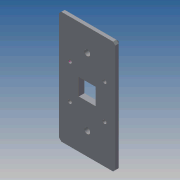
# Autodesk Inventor part: nema y axis cover
Saved by Autodesk Inventor 2015 (Build 190159000, 159)
## iProperties
Created: 2015-10-11
Part Number: nema y axis cover
Material: Generic
Document SubType Name: Modeling
Designer: Solomon
Density: 1 g/cm^3
Appearance: Default
Author: Solomon
Autodesk Inventor part; units mm, degrees
ref_plane "YZ Plane" through (0, 0, 0) normal (1, 0, 0) x (0, 1, 0)
ref_plane "XZ Plane" through (0, 0, 0) normal (0, 1, 0) x (-1, 0, 0)
ref_plane "XY Plane" through (0, 0, 0) normal (0, 0, 1) x (1, 0, 0)
sketch "Sketch1" plane through (0, 0, 0) normal (0, 1, 0) x (-1, 0, 0)
  point P0 (0, 0)
sketch "Sketch2" plane through (0, 0, 0) normal (0, 1, 0) x (-1, 0, 0)
  line L0 (0, 0) -> (-31, 0)
  line L1 (-31, -1.65) -> (-31, -29.35)
  line L2 (-31, -31) -> (0, -31)
  line L3 (0, -29.35) -> (0, -1.65)
  circle A0 centre (0, 0) radius 1.65
  circle A1 centre (0, -31) radius 1.65
  circle A2 centre (-31, -31) radius 1.65
  circle A3 centre (-31, 0) radius 1.65
  line L4 (-15.5, -15.5) -> (-15.5, -45.5)
  line L5 (-15.5, 0) -> (-15.5, 14.5)
  circle A4 centre (-15.5, 14.5) radius 2.65
  circle A5 centre (-15.5, -45.5) radius 2.65
  line L6 (9.5, 34.5) -> (-40.5, 34.5)
  line L7 (-40.5, 34.5) -> (-40.5, -65.5)
  line L8 (-40.5, -65.5) -> (9.5, -65.5)
  line L9 (9.5, -65.5) -> (9.5, 34.5)
  line L10 (9.5, 34.5) -> (-40.5, -65.5) construction
  line L11 (-40.5, 34.5) -> (9.5, -65.5) construction
  line L12 (-8, -8) -> (-23, -8)
  line L13 (-23, -8) -> (-23, -23)
  line L14 (-23, -23) -> (-8, -23)
  line L15 (-8, -23) -> (-8, -8)
  line L16 (-8, -8) -> (-23, -23) construction
  line L17 (-23, -8) -> (-8, -23) construction
  dimension "d2" = 3.3
  dimension "d3" = 3.3
  dimension "d4" = 3.3
  dimension "d5" = 3.3
  dimension "d0" = 31
  dimension "d1" = 31
  dimension "d6" = 30
  dimension "d7" = 30
  dimension "d8" = 5.3
  dimension "d9" = 5.3
  dimension "d10" = 50
  dimension "d11" = 100
  dimension "d12" = 15
  dimension "d13" = 15
  constraints: 36 end point, 6 coincident, 6 parallel, 5 midpoint, 4 perpendicular, 4 vertical alignment, 3 horizontal, 2 centre point, 1 vertical, 8 other
  measures "d0" distance of L2.end L2.start
  measures "d1" distance of L2.start L0.end
  measures "d6" distance of L4.start L4.end
  measures "d7" distance of L4.start L5.end
  measures "d8" diameter of A4
  measures "d9" diameter of A5
  measures "d10" distance of L8.end L7.end
  measures "d11" distance of L7.end L6.end
  measures "d12" distance of L14.end L13.end
  measures "d13" distance of L13.end L12.end
extrude "Extrusion1" add sketch "Sketch2" along normal blind 5 contours L0 A0 L3 A1 L2 A2 L1 A3 | L9 L8 L7 L6
chamfer "Chamfer1" distance 2 angle 45 8 edges at (40.5, 2.5, 34.5) (40.5, 2.5, -65.5) (-9.5, 2.5, -65.5) (-9.5, 2.5, 34.5) (40.5, 5, -15.5) (15.5, 5, -65.5) (-9.5, 5, -15.5) (15.5, 5, 34.5)
body "Solid1"
